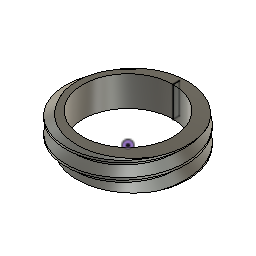
For13mmThreadM20x2.5-5mmTall v2 (Autodesk Fusion 360 design; units mm, degrees)
Autodesk Fusion 360 part; units mm, degrees
note: some values were not read from the file. Chosen so that the rebuilt part matches the saved one: that a step has no effect; where a thread starts. Set by a fixed rule: which sketch regions a step uses.
sketch "Sketch1" plane through (0, 0, 0) normal (1, 0, 0) x (0, 1, 0)
  line L0 (7.5, 0) -> (7.5, 5)
  line L1 (8.5, 5) -> (8.5, 0)
  line L2 (8.5, 0) -> (7.5, 0)
  line L3 (7.5, 5) -> (8.5, 5)
  dimension "d1" = 1
  dimension "d2" = 5
  dimension "d4" = 5
  dimension "d5" = 7.5
  constraint horizontal L2
  constraint coincident origin L2
  constraint horizontal L3
  constraint vertical L0
  constraint vertical L1
  measures "d1" distance of L0.start L1.end
  measures "d2" distance of L0.start L0.end
  measures "d4" distance of L1.start L1.end
  measures "d5" distance of origin L0.start
revolve "Revolve1" add sketch "Sketch1" angle 360 about axis through (0, 0, 1.75) along (0, 0, 1)
thread "Thread1" "ANSI Metric M Profile 20.0 M20x2.5 6g" major diameter 19.7905 minor diameter 16.938 pitch 2.5 angle 60 modelled right hand crest width 0.36 on face at (0.4237, 8.4894, 3.3333) crest through (0, 9.8953, 0.625)
extrude "Extrude4" [no effect]
